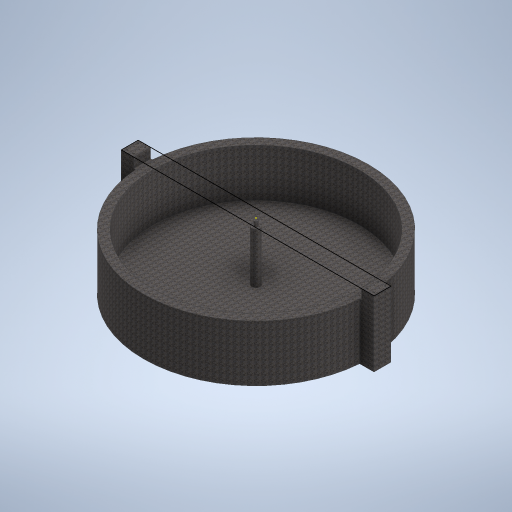
# Autodesk Inventor part: Vasca
Saved by Autodesk Inventor 2024.2 (Build 282272000, 272)
## iProperties
Created: 2024-03-18
Part Number: Vasca
Material: Concrete
Document SubType Name: Modeling
Designer: feder
Density: 2.40731 g/cm^3
Appearance: Exposed Aggregate - Coarse
Mass: 7.19804e+07 g
Surface Area: 1.98507e+06 cm^2
Volume: 2.99007e+07 cm^3
Author: feder
Autodesk Inventor part; units mm, degrees
ref_plane "YZ Plane" through (0, 0, 0) normal (1, 0, 0) x (0, 1, 0)
ref_plane "XZ Plane" through (0, 0, 0) normal (0, 1, 0) x (-1, 0, 0)
ref_plane "XY Plane" through (0, 0, 0) normal (0, 0, 1) x (1, 0, 0)
sketch "Sketch1" plane through (0, 0, 0) normal (0, 1, 0) x (-1, 0, 0)
  circle A0 centre (0, 0) radius 4000 construction
  circle A1 centre (0, 0) radius 4000
  circle A2 centre (0, 0) radius 3675
  dimension "d0" = 8000
  dimension "d29" = 7350
  dimension "d30" = 8000
  constraints: 3 centre point, 1 coincident
  measures "d0" diameter of A0
  measures "d29" diameter of A2
  measures "d30" diameter of A1
extrude "Extrusion1" add sketch "Sketch1" along normal blind 1700
sketch "Sketch5" plane through (0, 0, 0) normal (0, -1, 0) x (1, 0, 0)
  circle A0 centre (0, 0) radius 4000
  dimension "d31" = 8000
  constraints: 1 centre point, 1 coincident
  measures "d31" diameter of A0
extrude "Extrusion5" add sketch "Sketch5" along normal blind 300
sketch "Sketch6" plane through (0, 0, 0) normal (0, 1, 0) x (1, 0, 0)
  circle A0 centre (0, 0) radius 150
  dimension "d15" = 300
  constraints: 1 centre point, 1 coincident
  measures "d15" diameter of A0
extrude "Extrusion6" add sketch "Sketch6" along normal blind 1805
sketch "Sketch7" plane through (0, 1805, 0) normal (0, 1, 0) x (1, 0, 0)
  circle A0 centre (0, 0) radius 65
  dimension "d18" = 130
  constraints: 1 centre point, 1 coincident
  measures "d18" diameter of A0
extrude "Extrusion7" add sketch "Sketch7" along normal blind 177
sketch "Sketch8" plane through (0, 1700, 0) normal (0, 1, 0) x (1, 0, 0)
  circle A0 centre (0, 0) radius 65 projected
  circle A1 centre (0, 0) radius 4000
  circle A2 centre (0, 0) radius 4500
  line L0 (3988.7341, -300) -> (4500, -300)
  line L1 (4500, -300) -> (4500, 300)
  line L2 (4500, 300) -> (3988.7341, 300)
  line L3 (4000, 300) -> (4000, -300)
  line L4 (4000, -300) -> (4500, 300) construction
  line L5 (4500, -300) -> (4000, 300) construction
  line L6 (0, 4500) -> (0, -5103.1646) construction
  line L7 (-3988.7341, -300) -> (-4500, -300)
  line L8 (-4500, -300) -> (-4500, 300)
  line L9 (-4500, 300) -> (-3988.7341, 300)
  line L10 (-4000, 300) -> (-4000, -300)
  line L11 (-4000, -300) -> (-4500, 300) construction
  line L12 (-4500, -300) -> (-4000, 300) construction
  point P0 (4250, 0)
  point P1 (-4250, 0)
  point P2 (-3988.7341, -300)
  point P3 (-3988.7341, 300)
  dimension "d35" = 8000
  dimension "d40" = 500
  dimension "d41" = 600
  constraints: 26 end point, 7 symmetric about line, 4 midpoint, 4 point on line, 3 vertical, 2 parallel, 2 point on circle, 1 centre point, 1 coincident, 1 horizontal, 1 perpendicular, 1 tangent, 1 vertical alignment, 2 other
  measures "d35" diameter of A1
  measures "d41" distance of L1.end L0.end
extrude "Extrusion8" add sketch "Sketch8" against normal up to surface (2000 mm away) contours L3 L0 A1 | A1 L2 L3 | L3 L2 A2 L0 | A1 L10 L9 | L7 L10 A1 | L2 L1 A2 | A2 L1 L0 | L10 L7 A2 L9 | A2 L8 L9 | L7 L8 A2
sketch "Sketch10" plane through (0, 1700, 0) normal (0, 1, 0) x (1, 0, 0)
  line L0 (-3988.7341, 300) -> (-4500, 300) projected
  line L1 (-4500, -300) -> (-3988.7341, -300) projected
  line L2 (-4500, 300) -> (-4050, 300)
  line L3 (-4050, 300) -> (-4050, -300)
  line L4 (-4050, -300) -> (-4500, -300)
  line L5 (-4500, -300) -> (-4500, 300)
  line L6 (4500, -300) -> (4500, 300) projected
  line L7 (4500, 300) -> (4050, 300)
  line L8 (4050, 300) -> (4050, -300)
  line L9 (4050, -300) -> (4500, -300)
  line L10 (4500, -300) -> (4500, 300)
  point P0 (0, 0)
  point P1 (-4050, 300)
  point P2 (-4050, 300)
  dimension "d43" = 450
  dimension "d44" = 450
  constraints: 16 end point, 4 parallel, 2 horizontal, 2 perpendicular, 2 point on line
  measures "d43" distance of L3.end L4.end
  measures "d44" distance of L9.end L8.end
extrude "Extrusion10" add sketch "Sketch10" along normal blind 352
sketch "Sketch11" plane through (0, 2052, 0) normal (0, 1, 0) x (1, 0, 0)
  line L0 (-4500, 300) -> (-4500, -300) projected
  line L1 (4050, -300) -> (4500, -300) projected
  line L2 (-4500, 300) -> (4500, 300)
  line L3 (4500, 300) -> (4500, -300)
  line L4 (4500, -300) -> (-4500, -300)
  line L5 (-4500, -300) -> (-4500, 300)
  point P0 (0, 0)
  constraints: 8 end point, 2 parallel, 1 horizontal, 1 perpendicular
sketch "Sketch12" plane through (0, 2052, 0) normal (0, 1, 0) x (1, 0, 0)
  line L0 (-3988.7341, 300) -> (-4500, 300) projected
  line L1 (-4050, -300) -> (-3988.7341, -300) projected
  line L2 (-4500, 300) -> (-4050, 300)
  line L3 (-4050, 300) -> (-4050, -300)
  line L4 (-4050, -300) -> (-4500, -300)
  line L5 (-4500, -300) -> (-4500, 300)
  line L6 (-4400, 200) -> (-4150, 200)
  line L7 (-4150, 200) -> (-4150, -200)
  line L8 (-4150, -200) -> (-4400, -200)
  line L9 (-4400, -200) -> (-4400, 200)
  line L10 (0, 5520.4095) -> (0, -5368.8003) construction
  line L11 (3988.7341, 300) -> (4500, 300)
  line L12 (4050, -300) -> (3988.7341, -300)
  line L13 (4500, 300) -> (4050, 300)
  line L14 (4050, 300) -> (4050, -300)
  line L15 (4050, -300) -> (4500, -300)
  line L16 (4500, -300) -> (4500, 300)
  line L17 (4400, 200) -> (4150, 200)
  line L18 (4150, 200) -> (4150, -200)
  line L19 (4150, -200) -> (4400, -200)
  line L20 (4400, -200) -> (4400, 200)
  circle A0 centre (-4400, 200) radius 25
  circle A1 centre (-4150, 200) radius 25
  circle A2 centre (-4400, -200) radius 25
  circle A3 centre (-4150, -200) radius 25
  circle A4 centre (4150, 200) radius 25
  circle A5 centre (4400, 200) radius 25
  circle A6 centre (4150, -200) radius 25
  circle A7 centre (4400, -200) radius 25
  point P0 (0, 0)
  dimension "d47" = 100
  dimension "d48" = 50
  dimension "d49" = 50
  dimension "d50" = 50
  dimension "d51" = 50
  dimension "d52" = 50
  dimension "d53" = 50
  dimension "d54" = 50
  dimension "d55" = 50
  constraints: 38 end point, 10 symmetric about line, 8 centre point, 8 coincident, 4 parallel, 2 perpendicular, 1 horizontal, 1 vertical, 3 other
  measures "d47" distance between parallel lines of L5 L9
  measures "d48" diameter of A0
  measures "d49" diameter of A1
  measures "d50" diameter of A2
  measures "d51" diameter of A3
  measures "d52" diameter of A4
  measures "d53" diameter of A5
  measures "d54" diameter of A6
  measures "d55" diameter of A7
extrude "Extrusion11" cut sketch "Sketch12" against normal blind 100 contours L9 A0 L6 | L6 A0 L9 | A1 L7 L6 | L6 L7 A1 | A2 L8 L9 | L9 L8 A2 | A3 L8 L7 | L7 L8 A3 | A4 L18 L17 | L17 L18 A4 | A5 L20 L17 | L17 L20 A5 | A6 L19 L18 | L18 L19 A6 | A7 L19 L20 | L20 L19 A7
body "Solid1"
